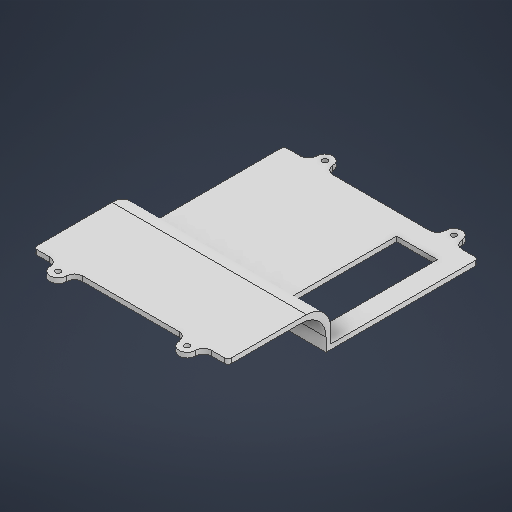
# Autodesk Inventor part: top
Saved by Autodesk Inventor 2026.1 (Build 301233020, 233B)
## iProperties
Created: 2026-07-01
Part Number: top
Material: Generic
Document SubType Name: Modeling
Designer: Asus
Density: 1 g/cm^3
Appearance: Default
Author: Asus
Autodesk Inventor part; units mm, degrees
ref_plane "YZ Plane" through (0, 0, 0) normal (1, 0, 0) x (0, 1, 0)
ref_plane "XZ Plane" through (0, 0, 0) normal (0, 1, 0) x (-1, 0, 0)
ref_plane "XY Plane" through (0, 0, 0) normal (0, 0, 1) x (1, 0, 0)
sketch "Sketch1" plane through (0, 0, 0) normal (0, 1, 0) x (-1, 0, 0)
  line L0 (0, 0) -> (119, 0)
  line L1 (119, 0) -> (119, -90.25)
  line L2 (119, -90.25) -> (0, -90.25)
  line L3 (0, -90.25) -> (0, 0)
  dimension "d0" = 119
  dimension "d1" = 90.25
  constraints: 8 end point, 2 parallel, 1 horizontal, 1 perpendicular
  measures "d0" distance of L1.end L2.end
  measures "d1" distance of L0.end L1.end
extrude "Extrusion1" add sketch "Sketch1" along normal blind 3
sketch "Sketch2" plane through (-119, 0, 0) normal (0, 0, 1) x (1, 0, 0)
  line L0 (119, 0) -> (0, 0) projected
  line L1 (0, 0) -> (119, 0)
  line L2 (119, 0) -> (119, 23)
  line L3 (119, 23) -> (0, 23)
  line L4 (0, 23) -> (0, 0)
  dimension "d4" = 23
  constraints: 8 end point, 2 parallel, 1 horizontal, 1 perpendicular
  measures "d4" distance of L2.end L1.end
extrude "Extrusion2" add sketch "Sketch2" along normal blind 3
sketch "Sketch3" plane through (-119, 23, 0) normal (0, 1, 0) x (1, 0, 0)
  line L0 (119, 0) -> (119, 90.25) projected
  line L1 (119, 0) -> (0, 0)
  line L2 (0, 0) -> (0, -63)
  line L3 (0, -63) -> (119, -63)
  line L4 (119, -63) -> (119, 0)
  dimension "d7" = 119
  dimension "d8" = 63
  constraints: 8 end point, 2 parallel, 1 horizontal, 1 perpendicular
  measures "d7" distance of L3.end L2.end
  measures "d8" distance of L2.end L1.end
extrude "Extrusion3" add sketch "Sketch3" along normal blind 3
fillet "Fillet1" radius 15 2 edges at (-59.5, 26, 0) (-59.5, 23, 3)
sketch "Sketch4" plane through (0, 0, -90.25) normal (0, 0, -1) x (-1, 0, 0)
  line L0 (0, 3) -> (119, 3) projected
  line L1 (15, 3) -> (25, 3)
  line L2 (25, 3) -> (25, 0)
  line L3 (25, 0) -> (15, 0)
  line L4 (15, 0) -> (15, 3)
  line L5 (0, 0) -> (0, 3) projected
  line L6 (94, 3) -> (104, 3)
  line L7 (104, 3) -> (104, 0)
  line L8 (104, 0) -> (94, 0)
  line L9 (94, 0) -> (94, 3)
  line L10 (119, 0) -> (119, 3) projected
  point P0 (15, 1.5)
  point P1 (0, 1.5)
  point P2 (104, 1.5)
  point P3 (119, 1.5)
  dimension "d12" = 10
  dimension "d13" = 3
  dimension "d14" = 15
  dimension "d15" = 10
  dimension "d16" = 3
  dimension "d17" = 15
  constraints: 16 end point, 4 midpoint, 4 parallel, 2 horizontal, 2 perpendicular, 2 point on line
  measures "d12" distance of L2.end L3.end
  measures "d13" distance of L1.end L2.end
  measures "d14" distance of point (15, 1.5) point (0, 1.5)
  measures "d15" distance of L7.end L8.end
  measures "d16" distance of L6.end L7.end
  measures "d17" distance of point (104, 1.5) point (119, 1.5)
extrude "Extrusion4" add sketch "Sketch4" along normal blind 10
sketch "Sketch5" plane through (-119, 23, 63) normal (0, 0, 1) x (1, 0, 0)
  line L0 (0, 3) -> (119, 3) projected
  line L1 (15, 3) -> (25, 3)
  line L2 (25, 3) -> (25, 0)
  line L3 (25, 0) -> (15, 0)
  line L4 (15, 0) -> (15, 3)
  line L5 (94, 3) -> (104, 3)
  line L6 (104, 3) -> (104, 0)
  line L7 (104, 0) -> (94, 0)
  line L8 (94, 0) -> (94, 3)
  line L9 (0, 0) -> (0, 3) projected
  line L10 (119, 0) -> (119, 3) projected
  point P0 (119, -23)
  point P1 (15, 1.5)
  point P2 (0, 1.5)
  point P3 (119, 1.5)
  point P4 (104, 1.5)
  point P5 (104, 3)
  point P6 (94, 3)
  point P7 (25, 3)
  dimension "d20" = 10
  dimension "d21" = 3
  dimension "d22" = 10
  dimension "d23" = 3
  dimension "d24" = 15
  dimension "d25" = 15
  constraints: 16 end point, 4 midpoint, 4 parallel, 2 horizontal, 2 perpendicular, 2 point on line
  measures "d20" distance of L2.end L3.end
  measures "d21" distance of L1.end L2.end
  measures "d22" distance of L6.end L7.end
  measures "d23" distance of L5.end L6.end
  measures "d24" distance of point (15, 1.5) point (0, 1.5)
  measures "d25" distance of point (119, 1.5) point (104, 1.5)
extrude "Extrusion5" add sketch "Sketch5" along normal blind 10
sketch "Sketch6" plane through (-119, 26, 0) normal (0, 1, 0) x (1, 0, 0)
  circle A0 centre (20, -68) radius 1.65
  line L0 (15, -63) -> (15, -73) projected
  line L1 (25, -73) -> (15, -73) projected
  circle A1 centre (99, -68) radius 1.65
  line L2 (104, -73) -> (94, -73) projected
  line L3 (94, -63) -> (94, -73) projected
  point P0 (119, 0)
  point P1 (15, -68)
  point P2 (99, -73)
  dimension "d28" = 3.3
  dimension "d29" = 5
  dimension "d30" = 5
  dimension "d31" = 3.3
  dimension "d32" = 5
  dimension "d33" = 5
  constraints: 2 centre point, 2 midpoint
  measures "d28" diameter of A0
  measures "d29" distance of A0.centre point (15, -68)
  measures "d30" distance from line of A0.centre L1
  measures "d31" diameter of A1
  measures "d32" distance of point (99, -73) A1.centre
  measures "d33" distance from line of L3 A1.centre
extrude "Extrusion6" cut sketch "Sketch6" against normal blind 5
sketch "Sketch7" plane through (0, 3, 0) normal (0, 1, 0) x (1, 0, 0)
  circle A0 centre (-99, 95.25) radius 1.65
  circle A1 centre (-20, 95.25) radius 1.65
  line L0 (-104, 90.25) -> (-104, 100.25) projected
  line L1 (-104, 100.25) -> (-94, 100.25) projected
  line L2 (-25, 90.25) -> (-25, 100.25) projected
  line L3 (-25, 100.25) -> (-15, 100.25) projected
  point P0 (0, 0)
  point P1 (-104, 95.25)
  dimension "d36" = 3.3
  dimension "d37" = 3.3
  dimension "d38" = 5
  dimension "d39" = 5
  dimension "d40" = 5
  dimension "d41" = 5
  constraints: 2 centre point, 1 midpoint
  measures "d36" diameter of A0
  measures "d37" diameter of A1
  measures "d38" distance of point (-104, 95.25) A0.centre
  measures "d39" distance from line of L1 A0.centre
  measures "d40" distance from line of L2 A1.centre
  measures "d41" distance from line of L3 A1.centre
extrude "Extrusion7" cut sketch "Sketch7" against normal blind 5
fillet "Fillet2" radius 5 16 edges at (-15, 24.5, 73) (-15, 24.5, 63) (-25, 24.5, 73) (-25, 24.5, 63) (-104, 24.5, 63) (-104, 24.5, 73) (-94, 24.5, 73) (-94, 24.5, 63) (-15, 1.5, -90.25) (-15, 1.5, -100.25) (-25, 1.5, -100.25) (-25, 1.5, -90.25) (-94, 1.5, -100.25) (-104, 1.5, -100.25) (-104, 1.5, -90.25) (-94, 1.5, -90.25)
fillet "Fillet3" radius 2 4 edges at (0, 1.5, -90.25) (-119, 1.5, -90.25) (-119, 24.5, 63) (0, 24.5, 63)
sketch "Sketch8" plane through (0, 3, 0) normal (0, 1, 0) x (1, 0, 0)
  line L0 (-37, 6.25) -> (-12, 6.25)
  line L1 (-12, 6.25) -> (-12, 77.25)
  line L2 (-12, 77.25) -> (-37, 77.25)
  line L3 (-37, 77.25) -> (-37, 6.25)
  line L4 (0, 0) -> (0, 88.25) projected
  line L5 (-2, 90.25) -> (-10, 90.25) projected
  dimension "d46" = 25
  dimension "d47" = 71
  dimension "d48" = 12
  dimension "d49" = 13
  constraints: 8 end point, 2 parallel, 1 horizontal, 1 perpendicular
  measures "d46" distance of L2.end L1.end
  measures "d47" distance of L1.end L0.end
  measures "d48" distance between parallel lines of L4 L1
  measures "d49" distance between parallel lines of L5 L2
extrude "Extrusion8" cut sketch "Sketch8" against normal blind 5
equation "\"d34\" = d30"
equation "\"d42\" = d30"
equation "\"d50\" = d30"
body "Solid1"
